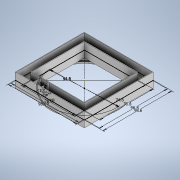
# Autodesk Inventor part: Part3
Saved by Autodesk Inventor 2022 (Build 260153000, 153)
## iProperties
Created: 2022-03-29
Part Number: Part3
Material: Generic
Document SubType Name: Modeling
Designer: Hajar
Density: 1 g/cm^3
Appearance: Default
Author: Hajar
Autodesk Inventor part; units mm, degrees
ref_plane "YZ Plane" through (0, 0, 0) normal (1, 0, 0) x (0, 1, 0)
ref_plane "XZ Plane" through (0, 0, 0) normal (0, 1, 0) x (-1, 0, 0)
ref_plane "XY Plane" through (0, 0, 0) normal (0, 0, 1) x (1, 0, 0)
sketch "Sketch1" plane through (0, 0, 0) normal (0, 1, 0) x (-1, 0, 0)
  line L0 (49.3, -49.3) -> (-49.3, -49.3)
  line L1 (-49.3, -49.3) -> (-49.3, 49.3)
  line L2 (-49.3, 49.3) -> (49.3, 49.3)
  line L3 (49.3, 49.3) -> (49.3, -49.3)
  line L4 (49.3, -49.3) -> (-49.3, 49.3) construction
  line L5 (-49.3, -49.3) -> (49.3, 49.3) construction
  line L6 (48.4, -48.4) -> (-48.4, -48.4)
  line L7 (-48.4, -48.4) -> (-48.4, 48.4)
  line L8 (-48.4, 48.4) -> (48.4, 48.4)
  line L9 (48.4, 48.4) -> (48.4, -48.4)
  line L10 (48.4, -48.4) -> (-48.4, 48.4) construction
  line L11 (-48.4, -48.4) -> (48.4, 48.4) construction
  line L12 (38.4, -38.4) -> (-38.4, -38.4)
  line L13 (-38.4, -38.4) -> (-38.4, 38.4)
  line L14 (-38.4, 38.4) -> (38.4, 38.4)
  line L15 (38.4, 38.4) -> (38.4, -38.4)
  line L16 (38.4, -38.4) -> (-38.4, 38.4) construction
  line L17 (-38.4, -38.4) -> (38.4, 38.4) construction
  line L18 (37.4, -37.4) -> (-37.4, -37.4)
  line L19 (-37.4, -37.4) -> (-37.4, 37.4)
  line L20 (-37.4, 37.4) -> (37.4, 37.4)
  line L21 (37.4, 37.4) -> (37.4, -37.4)
  line L22 (37.4, -37.4) -> (-37.4, 37.4) construction
  line L23 (-37.4, -37.4) -> (37.4, 37.4) construction
  line L24 (24.3286, 38.4) -> (24.3286, 48.4)
  line L25 (24.3286, 38.4) -> (23.3286, 38.4)
  line L26 (23.3286, 38.4) -> (23.3286, 48.4)
  line L27 (24.3286, 48.4) -> (23.3286, 48.4)
  circle A0 centre (17.6595, 43.4) radius 3.4806
  line L28 (12.8049, 38.4) -> (12.8049, 41.4)
  line L29 (12.8049, 41.4) -> (11.8049, 41.4)
  line L30 (11.8049, 41.4) -> (11.8049, 38.4)
  line L31 (12.8049, 48.4) -> (12.8049, 45.4)
  line L32 (12.8049, 45.4) -> (11.8049, 45.4)
  line L33 (11.8049, 45.4) -> (11.8049, 48.4)
  point P0 (0, 0)
  dimension "d0" = 98.6
  dimension "d1" = 98.6
  dimension "d2" = 96.8
  dimension "d3" = 96.8
  dimension "d4" = 76.8
  dimension "d5" = 76.8
  dimension "d6" = 74.8
  dimension "d7" = 74.8
  dimension "d8" = 10
  dimension "d9" = 1
  dimension "d10" = 3
  dimension "d11" = 1
  dimension "d12" = 3
  constraints: 68 end point, 12 point on line, 10 perpendicular, 8 midpoint, 8 parallel, 4 horizontal, 1 centre point, 1 vertical
  measures "d0" distance of L1.end L2.end
  measures "d1" distance of L0.end L1.end
  measures "d2" distance of L7.end L8.end
  measures "d3" distance of L6.end L7.end
  measures "d4" distance of L13.end L14.end
  measures "d5" distance of L12.end L13.end
  measures "d6" distance of L19.end L20.end
  measures "d7" distance of L18.end L19.end
  measures "d8" distance of L24.start L24.end
  measures "d9" distance of L24.start L25.end
  measures "d10" distance of L28.start L28.end
  measures "d11" distance of L28.end L29.end
  measures "d12" distance of L31.start L31.end
extrude "Extrusion1" add sketch "Sketch1" along normal mid plane 20 contours L0 L1 L2 L3 | L6 L7 L8 L33 L32 L31 L26 L14 L28 L29 L30 L13 L12 L15 L24 L9 | L24 L14 L26 L8 | L8 L31 L32 L33 | L14 L15 L12 L13 | L14 L30 L29 L28 | L18 L19 L20 L21 | A0
extrude "Extrusion2" cut sketch "Sketch1" along normal mid plane 29.525 contours L18 L19 L20 L21
extrude "Extrusion3" cut sketch "Sketch1" along normal blind 29.525 and the other way blind 8 contours L6 L7 L8 L33 L32 L31 L26 L14 L28 L29 L30 L13 L12 L15 L24 L9
extrude "Extrusion4" cut sketch "Sketch1" along normal blind 29.525 and the other way blind 14.763 contours A0
sketch "Sketch2" plane through (0, -10, 0) normal (0, -1, 0) x (1, 0, 0)
  arc A0 (40.1076, -27.0913) -> (-15.2678, 45.9288) centre (0, 0) ccw
  arc A1 (-14.6167, 45.09) -> (-14.6288, 45.0861) centre (0, 0) ccw
  circle A2 centre (-17.6595, 43.4) radius 3.4806 projected
  line L0 (-14.6288, 45.0861) -> (-14.5793, 45.0208)
  circle A3 centre (0, 0) radius 47.4
  arc A4 (-15.2678, 45.9288) -> (-21.1372, 43.5405) centre (0, 0) ccw
  circle A5 centre (0, 0) radius 48.4
  arc A6 (-14.5793, 45.0208) -> (-14.6167, 45.09) centre (-17.6595, 43.4) ccw
  arc A7 (-15.2678, 45.9288) -> (-21.1372, 43.5405) centre (-17.6595, 43.4) ccw
  point P0 (-14.6167, 45.09)
  point P1 (-15.2678, 45.9288)
  point P2 (-14.6167, 45.09)
  dimension "d25" = 96.8
  dimension "d26" = 94.8
  constraints: 19 point on circle, 7 centre point, 6 coincident, 3 concentric, 2 end point, 1 point on line
  measures "d25" diameter of A0
  measures "d26" diameter of A1
sketch "Sketch3" plane through (0, -10, 0) normal (0, -1, 0) x (1, 0, 0)
  arc A0 (-21.1372, 43.5405) -> (-15.2678, 45.9288) centre (0, 0) ccw projected
  line L0 (37.4, -37.4) -> (37.4, 37.4) projected
  line L1 (37.4, -29.1204) -> (37.4, -30.7213) projected
  line L2 (37.4, -30.7213) -> (37.4, -37.4)
  line L3 (37.4, -37.4) -> (-37.4, -37.4) projected
  line L4 (37.4, -37.4) -> (30.7213, -37.4)
  arc A1 (-37.4, -30.7213) -> (-30.7213, -37.4) centre (0, 0) ccw projected
  line L5 (-37.4, -37.4) -> (-30.7213, -37.4)
  arc A2 (-37.4, 30.7213) -> (-37.4, -30.7213) centre (0, 0) ccw projected
  line L6 (-37.4, -37.4) -> (-37.4, -30.7213)
  line L7 (-37.4, 37.4) -> (-37.4, -37.4) projected
  line L8 (-37.4, 30.7213) -> (-37.4, 37.4)
  line L9 (-37.4, 37.4) -> (37.4, 37.4) projected
  line L10 (-37.4, 37.4) -> (-30.7213, 37.4)
  arc A3 (37.4, 30.7213) -> (30.7213, 37.4) centre (0, 0) ccw projected
  line L11 (37.4, 37.4) -> (37.4, -37.4) projected
  line L12 (37.4, 30.7213) -> (37.4, 37.4)
  line L13 (-37.4, 37.4) -> (37.4, 37.4) projected
  line L14 (37.4, 37.4) -> (30.7213, 37.4)
  arc A4 (30.7213, -37.4) -> (37.4, -30.7213) centre (0, 0) ccw
  arc A5 (-37.4, -30.7213) -> (-30.7213, -37.4) centre (0, 0) ccw
  arc A6 (37.4, 30.7213) -> (30.7213, 37.4) centre (0, 0) ccw
  arc A7 (-30.7213, 37.4) -> (-37.4, 30.7213) centre (0, 0) ccw
  point P0 (37.4, 30.7213)
  point P1 (37.4, -30.7213)
  constraints: 16 end point, 8 point on circle, 4 centre point, 4 collinear, 2 perpendicular, 2 point on line, 1 coincident, 1 horizontal, 1 vertical, 1 other
extrude "Extrusion6" add sketch "Sketch3" against normal blind 0.175 contours A0 L7 L9 | L9 L0 A0 | A0 L3 L6 | L0 L3 A0
extrude "Extrusion8" add sketch "Sketch2" against normal blind 0.175 contours A2 A4
extrude "Extrusion9" add sketch "Sketch2" along normal blind 3 contours A5 A2 A3 A0 | A4 A2 A1 A3
body "Solid1"
